Autodesk Inventor part; units mm, degrees
(part 6 of 6)
  arc A568 (-14.0614, 14.9173) -> (-13.8819, 14.463) centre (-6.919, 17.4773) ccw projected
  arc A569 (-13.7681, 15.1885) -> (-14.0614, 14.9173) centre (0, 0) ccw projected
  arc A570 (-13.3293, 14.9739) -> (-13.7681, 15.1885) centre (-16.8806, 8.2689) ccw projected
  arc A571 (-12.9866, 14.7786) -> (-13.3293, 14.9739) centre (-16.3285, 9.3114) ccw projected
  arc A572 (-12.7266, 14.609) -> (-12.9866, 14.7786) centre (-15.7361, 10.2805) ccw projected
  arc A573 (-12.4383, 14.8553) -> (-12.7266, 14.609) centre (0, 0) ccw projected
  arc A574 (-12.5651, 15.1386) -> (-12.4383, 14.8553) centre (-7.6922, 17.1506) ccw projected
  arc A575 (-12.7043, 15.5076) -> (-12.5651, 15.1386) centre (-6.6424, 17.5841) ccw projected
  arc A576 (-12.8477, 15.9746) -> (-12.7043, 15.5076) centre (-5.5264, 17.9663) ccw projected
  arc A577 (-12.534, 16.2219) -> (-12.8477, 15.9746) centre (0, 0) ccw projected
  arc A578 (-12.1134, 15.9735) -> (-12.534, 16.2219) centre (-16.1798, 9.5679) ccw projected
  arc A579 (-11.7871, 15.752) -> (-12.1134, 15.9735) centre (-15.5476, 10.5638) ccw projected
  arc A580 (-11.5412, 15.5625) -> (-11.7871, 15.752) centre (-14.881, 11.4834) ccw projected
  arc A581 (-11.2344, 15.7854) -> (-11.5412, 15.5625) centre (0, 0) ccw projected
  arc A582 (-11.3386, 16.0778) -> (-11.2344, 15.7854) centre (-6.3229, 17.7012) ccw projected
  arc A583 (-11.4485, 16.4566) -> (-11.3386, 16.0778) centre (-5.2423, 18.051) ccw projected
  arc A584 (-11.5547, 16.9334) -> (-11.4485, 16.4566) centre (-4.0998, 18.3445) ccw projected
  arc A585 (-11.2226, 17.1553) -> (-11.5547, 16.9334) centre (0, 0) ccw projected
  arc A586 (-10.8227, 16.8747) -> (-11.2226, 17.1553) centre (-15.3792, 10.8078) ccw projected
  arc A587 (-10.5148, 16.6282) -> (-10.8227, 16.8747) centre (-14.6708, 11.7511) ccw projected
  arc A588 (-10.2846, 16.42) -> (-10.5148, 16.6282) centre (-13.9341, 12.6156) ccw projected
  arc A589 (-9.9612, 16.6182) -> (-10.2846, 16.42) centre (0, 0) ccw projected
  arc A590 (-10.0422, 16.9178) -> (-9.9612, 16.6182) centre (-4.9146, 18.1428) ccw projected
  arc A591 (-10.122, 17.3041) -> (-10.0422, 16.9178) centre (-3.8099, 18.4067) ccw projected
  arc A592 (-10.1905, 17.7877) -> (-10.122, 17.3041) centre (-2.6478, 18.6096) ccw projected
  arc A593 (-9.842, 17.9829) -> (-10.1905, 17.7877) centre (0, 0) ccw projected
  arc A594 (-9.4654, 17.6718) -> (-9.842, 17.9829) centre (-14.4838, 11.9812) ccw projected
  arc A595 (-9.1778, 17.4019) -> (-9.4654, 17.6718) centre (-13.7036, 12.8659) ccw projected
  arc A596 (-8.9646, 17.1763) -> (-9.1778, 17.4019) centre (-12.9014, 13.6699) ccw projected
  arc A597 (-8.6267, 17.3485) -> (-8.9646, 17.1763) centre (0, 0) ccw projected
  arc A598 (-8.6839, 17.6536) -> (-8.6267, 17.3485) centre (-3.476, 18.4724) ccw projected
  arc A599 (-8.7331, 18.0449) -> (-8.6839, 17.6536) centre (-2.3539, 18.6488) ccw projected
  arc A600 (-8.7635, 18.5324) -> (-8.7331, 18.0449) centre (-1.1796, 18.76) ccw projected
  arc A601 (-8.4007, 18.6997) -> (-8.7635, 18.5324) centre (0, 0) ccw projected
  arc A602 (-8.0497, 18.36) -> (-8.4007, 18.6997) centre (-13.4991, 13.0806) ccw projected
  arc A603 (-7.7842, 18.0684) -> (-8.0497, 18.36) centre (-12.6519, 13.9014) ccw projected
  arc A604 (-7.5893, 17.8267) -> (-7.7842, 18.0684) centre (-11.7891, 14.64) ccw projected
  arc A605 (-7.2389, 17.9719) -> (-7.5893, 17.8267) centre (0, 0) ccw projected
  arc A606 (-7.272, 18.2805) -> (-7.2389, 17.9719) centre (-2.0159, 18.6882) ccw projected
  arc A607 (-7.2904, 18.6745) -> (-7.272, 18.2805) centre (-0.8835, 18.776) ccw projected
  arc A608 (-7.2825, 19.1629) -> (-7.2904, 18.6745) centre (0.2959, 18.7947) ccw projected
  arc A609 (-6.9077, 19.3011) -> (-7.2825, 19.1629) centre (0, 0) ccw projected
  arc A610 (-6.5844, 18.9349) -> (-6.9077, 19.3011) centre (-12.4312, 14.0994) ccw projected
  arc A611 (-6.3425, 18.6234) -> (-6.5844, 18.9349) centre (-11.5222, 14.8512) ccw projected
  arc A612 (-6.1673, 18.3672) -> (-6.3425, 18.6234) centre (-10.6041, 15.5199) ccw projected
  arc A613 (-5.8066, 18.4844) -> (-6.1673, 18.3672) centre (0, 0) ccw projected
  arc A614 (-5.8154, 18.7947) -> (-5.8066, 18.4844) centre (-0.5434, 18.7888) ccw projected
  arc A615 (-5.8028, 19.1889) -> (-5.8154, 18.7947) centre (0.5924, 18.7875) ccw projected
  arc A616 (-5.7565, 19.6752) -> (-5.8028, 19.1889) centre (1.7696, 18.7136) ccw projected
  arc A617 (-5.372, 19.7836) -> (-5.7565, 19.6752) centre (0, 0) ccw projected
  arc A618 (-5.0785, 19.3932) -> (-5.372, 19.7836) centre (-11.2867, 15.0313) ccw projected
  arc A619 (-4.8618, 19.0636) -> (-5.0785, 19.3932) centre (-10.3215, 15.7095) ccw projected
  arc A620 (-4.7072, 18.7945) -> (-4.8618, 19.0636) centre (-9.3537, 16.304) ccw projected
  arc A621 (-4.3384, 18.883) -> (-4.7072, 18.7945) centre (0, 0) ccw projected
  arc A622 (-4.3228, 19.193) -> (-4.3384, 18.883) centre (0.9324, 18.7735) ccw projected
  arc A623 (-4.2793, 19.585) -> (-4.3228, 19.193) centre (2.0646, 18.6831) ccw projected
  arc A624 (-4.1951, 20.0662) -> (-4.2793, 19.585) centre (3.2324, 18.517) ccw projected
  arc A625 (-3.8033, 20.1441) -> (-4.1951, 20.0662) centre (0, 0) ccw projected
  arc A626 (-3.5413, 19.7318) -> (-3.8033, 20.1441) centre (-10.0726, 15.8705) ccw projected
  arc A627 (-3.3511, 19.3863) -> (-3.5413, 19.7318) centre (-9.0571, 16.4708) ccw projected
  arc A628 (-3.2181, 19.1059) -> (-3.3511, 19.3863) centre (-8.0457, 16.9876) ccw projected
  arc A629 (-2.8435, 19.1652) -> (-3.2181, 19.1059) centre (0, 0) ccw projected
  arc A630 (-2.8036, 19.473) -> (-2.8435, 19.1652) centre (2.4025, 18.6425) ccw projected
  arc A631 (-2.7295, 19.8604) -> (-2.8036, 19.473) centre (3.5241, 18.4635) ccw projected
  arc A632 (-2.6078, 20.3335) -> (-2.7295, 19.8604) centre (4.6753, 18.2064) ccw projected
  arc A633 (-2.2111, 20.3804) -> (-2.6078, 20.3335) centre (0, 0) ccw projected
  arc A634 (-1.9822, 19.9489) -> (-2.2111, 20.3804) centre (-8.7963, 16.6119) ccw projected
  arc A635 (-1.8197, 19.5895) -> (-1.9822, 19.9489) centre (-7.7369, 17.1307) ccw projected
  arc A636 (-1.7091, 19.2995) -> (-1.8197, 19.5895) centre (-6.6881, 17.5665) ccw projected
  arc A637 (-1.331, 19.3292) -> (-1.7091, 19.2995) centre (0, 0) ccw projected
  arc A638 (-1.2671, 19.633) -> (-1.331, 19.3292) centre (3.8577, 18.3965) ccw projected
  arc A639 (-1.1629, 20.0133) -> (-1.2671, 19.633) centre (4.9618, 18.1301) ccw projected
  arc A640 (-1.0044, 20.4754) -> (-1.1629, 20.0133) centre (6.0894, 17.7834) ccw projected
  arc A641 (-0.6052, 20.4911) -> (-1.0044, 20.4754) centre (0, 0) ccw projected
  arc A642 (-0.4109, 20.0429) -> (-0.6052, 20.4911) centre (-7.4658, 17.2508) ccw projected
  circle A643 centre (0, 0) radius 18.25 projected
  line L0 (-18.25, 0) -> (18.25, 0) construction
  arc A644 (-18.25, 2.5) -> (-18.25, -2.5) centre (-18.25, 0) ccw
  arc A645 (18.25, -2.5) -> (18.25, 2.5) centre (18.25, 0) ccw
  line L1 (0, 18.25) -> (0, -18.25) construction
  arc A646 (2.5, 18.25) -> (-2.5, 18.25) centre (0, 18.25) ccw
  arc A647 (-2.5, -18.25) -> (2.5, -18.25) centre (0, -18.25) ccw
  line L2 (-18.25, -2.5) -> (-18.078, -2.5)
  arc A648 (-14.7902, -2.5) -> (-2.5, -14.7902) centre (0, 0) ccw
  line L3 (-2.5, -18.078) -> (-2.5, -18.25)
  line L4 (2.5, -18.25) -> (2.5, -18.078)
  arc A649 (2.5, -14.7902) -> (14.7902, -2.5) centre (0, 0) ccw
  line L5 (18.078, -2.5) -> (18.25, -2.5)
  line L6 (18.25, 2.5) -> (18.078, 2.5)
  arc A650 (14.7902, 2.5) -> (2.5, 14.7902) centre (0, 0) ccw
  arc A651 (-2.5, 14.7902) -> (-14.7902, 2.5) centre (0, 0) ccw
  line L7 (2.5, 18.078) -> (2.5, 18.25)
  line L8 (-2.5, 18.25) -> (-2.5, 18.078)
  line L9 (-18.078, 2.5) -> (-18.25, 2.5)
  line L10 (-14.7902, -2.5) -> (-5.4544, -2.5)
  line L11 (-2.5, -5.4544) -> (-2.5, -14.7902)
  line L12 (2.5, -14.7902) -> (2.5, -5.4544)
  line L13 (-2.5, -2.5) -> (2.5, -2.5)
  line L14 (5.4544, -2.5) -> (14.7902, -2.5)
  line L15 (14.7902, 2.5) -> (5.4544, 2.5)
  line L16 (2.5, -2.5) -> (2.5, 2.5)
  line L17 (2.5, 5.4544) -> (2.5, 14.7902)
  line L18 (-2.5, 14.7902) -> (-2.5, 5.4544)
  line L19 (-2.5, 2.5) -> (-2.5, -2.5)
  line L20 (2.5, 2.5) -> (-2.5, 2.5)
  line L21 (-5.4544, 2.5) -> (-14.7902, 2.5)
  point P0 (148.5, -105)
  dimension "d20" = 5
  dimension "d21" = 5
  constraints: 50 parallel, 48 end point, 40 tangent, 20 point on circle, 8 centre point, 4 midpoint, 1 coincident, 1 horizontal, 1 vertical, 22 other
  measures "d20" diameter of A645
  measures "d21" diameter of A647
extrude "押し出し5" cut sketch "スケッチ5" against normal blind 10 contours A0 L17 A650 L15 | L14 A649 L12 A0 | A0 L21 A651 L18 | L11 A648 L10 A0
fillet "フィレット2" radius 1 8 edges at (163.2902, 102.5, 1.5) (163.2902, 107.5, 1.5) (151, 119.7902, 1.5) (146, 119.7902, 1.5) (146, 90.2098, 1.5) (151, 90.2098, 1.5) (133.7098, 102.5, 1.5) (133.7098, 107.5, 1.5)
fillet "フィレット3" radius 5 8 edges at (153.9544, 102.5, 1.5) (153.9544, 107.5, 1.5) (151, 99.5456, 1.5) (146, 99.5456, 1.5) (143.0456, 102.5, 1.5) (143.0456, 107.5, 1.5) (146, 110.4544, 1.5) (151, 110.4544, 1.5)
sketch "スケッチ6" plane through (0, 0, -5) normal (0, 0, -1) x (-1, 0, 0)
  circle A0 centre (-148.5, 105) radius 2 projected
  arc A1 (-149.1615, 109.6213) -> (-149.1982, 109.7586) centre (-149.7545, 109.5365) ccw projected
  arc A2 (-149.1982, 109.7586) -> (-149.402, 110.1264) centre (-150.7515, 109.1382) ccw projected
  arc A3 (-149.402, 110.1264) -> (-150.0725, 110.7903) centre (-151.8157, 108.3591) ccw projected
  arc A4 (-150.0725, 110.7903) -> (-150.6312, 110.6087) centre (-148.5, 105) ccw projected
  arc A5 (-150.6312, 110.6087) -> (-150.7841, 109.6791) centre (-147.7926, 109.6645) ccw projected
  arc A6 (-150.7841, 109.6791) -> (-150.7328, 109.2599) centre (-149.1115, 109.671) ccw projected
  arc A7 (-150.7328, 109.2599) -> (-150.6818, 109.1272) centre (-150.1522, 109.4071) ccw projected
  line L0 (-150.6818, 109.1272) -> (-150.4726, 108.7315) projected
  arc A8 (-150.6306, 108.0863) -> (-150.4726, 108.7315) centre (-150.9147, 108.4978) ccw projected
  arc A9 (-150.6306, 108.0863) -> (-150.7779, 107.9793) centre (-148.5, 105) ccw projected
  arc A10 (-151.4403, 108.0283) -> (-150.7779, 107.9793) centre (-151.0815, 108.3766) ccw projected
  line L1 (-151.4403, 108.0283) -> (-151.7519, 108.3493) projected
  arc A11 (-151.7519, 108.3493) -> (-151.8623, 108.4388) centre (-152.1817, 107.9321) ccw projected
  arc A12 (-151.8623, 108.4388) -> (-152.2451, 108.6171) centre (-152.7543, 107.0239) ccw projected
  arc A13 (-152.2451, 108.6171) -> (-153.1765, 108.759) centre (-153.1557, 105.7676) ccw projected
  arc A14 (-153.1765, 108.759) -> (-153.5209, 108.2848) centre (-148.5, 105) ccw projected
  arc A15 (-153.5209, 108.2848) -> (-153.0982, 107.4429) centre (-150.6695, 109.1895) ccw projected
  arc A16 (-153.0982, 107.4429) -> (-152.8103, 107.1339) centre (-151.7402, 108.4195) ccw projected
  arc A17 (-152.8103, 107.1339) -> (-152.691, 107.0565) centre (-152.4271, 107.5943) ccw projected
  line L2 (-152.691, 107.0565) -> (-152.2892, 106.8594) projected
  arc A18 (-152.0378, 106.2446) -> (-152.2892, 106.8594) centre (-152.5095, 106.4105) ccw projected
  arc A19 (-152.0378, 106.2446) -> (-152.094, 106.0715) centre (-148.5, 105) ccw projected
  arc A20 (-152.6588, 105.7217) -> (-152.094, 106.0715) centre (-152.5732, 106.2143) ccw projected
  line L3 (-152.6588, 105.7217) -> (-153.0995, 105.7982) projected
  arc A21 (-153.0995, 105.7982) -> (-153.2414, 105.8058) centre (-153.202, 105.2081) ccw projected
  arc A22 (-153.2414, 105.8058) -> (-153.656, 105.725) centre (-153.1314, 104.1367) ccw projected
  arc A23 (-153.656, 105.725) -> (-154.4929, 105.2923) centre (-152.7177, 102.8844) ccw projected
  arc A24 (-154.4929, 105.2923) -> (-154.4928, 104.7063) centre (-148.5, 105) ccw projected
  arc A25 (-154.4928, 104.7063) -> (-153.6559, 104.2736) centre (-152.7177, 107.1142) ccw projected
  arc A26 (-153.6559, 104.2736) -> (-153.2414, 104.1928) centre (-153.1313, 105.8619) ccw projected
  arc A27 (-153.2414, 104.1928) -> (-153.0993, 104.2004) centre (-153.2019, 104.7905) ccw projected
  line L4 (-153.0993, 104.2004) -> (-152.6585, 104.277) projected
  arc A28 (-152.0937, 103.9274) -> (-152.6585, 104.277) centre (-152.5728, 103.7844) ccw projected
  arc A29 (-152.0937, 103.9274) -> (-152.0374, 103.7543) centre (-148.5, 105) ccw projected
  arc A30 (-152.2887, 103.1394) -> (-152.0374, 103.7543) centre (-152.509, 103.5882) ccw projected
  line L5 (-152.2887, 103.1394) -> (-152.6903, 102.9423) projected
  arc A31 (-152.6903, 102.9423) -> (-152.8095, 102.8649) centre (-152.4263, 102.4046) ccw projected
  arc A32 (-152.8095, 102.8649) -> (-153.0974, 102.5559) centre (-151.7394, 101.5794) ccw projected
  arc A33 (-153.0974, 102.5559) -> (-153.5202, 101.714) centre (-150.6687, 100.8093) ccw projected
  arc A34 (-153.5202, 101.714) -> (-153.1756, 101.2399) centre (-148.5, 105) ccw projected
  arc A35 (-153.1756, 101.2399) -> (-152.2442, 101.3818) centre (-153.1548, 104.2313) ccw projected
  arc A36 (-152.2442, 101.3818) -> (-151.8614, 101.5601) centre (-152.7534, 102.9751) ccw projected
  arc A37 (-151.8614, 101.5601) -> (-151.7509, 101.6497) centre (-152.1808, 102.0668) ccw projected
  line L6 (-151.7509, 101.6497) -> (-151.4393, 101.9708) projected
  arc A38 (-150.7769, 102.0199) -> (-151.4393, 101.9708) centre (-151.0805, 101.6226) ccw projected
  arc A39 (-150.7769, 102.0199) -> (-150.6296, 101.913) centre (-148.5, 105) ccw projected
  arc A40 (-150.4715, 101.2678) -> (-150.6296, 101.913) centre (-150.9136, 101.5014) ccw projected
  line L7 (-150.4715, 101.2678) -> (-150.6805, 100.8723) projected
  arc A41 (-150.6805, 100.8723) -> (-150.7315, 100.7396) centre (-150.1509, 100.5924) ccw projected
  arc A42 (-150.7315, 100.7396) -> (-150.7828, 100.3204) centre (-149.1102, 100.3285) ccw projected
  arc A43 (-150.7828, 100.3204) -> (-150.6299, 99.3908) centre (-147.7913, 100.335) ccw projected
  arc A44 (-150.6299, 99.3908) -> (-150.0725, 99.2097) centre (-148.5, 105) ccw projected
  arc A45 (-150.0725, 99.2097) -> (-149.4024, 99.872) centre (-151.814, 101.6421) ccw projected
  arc A46 (-149.4024, 99.872) -> (-149.1975, 100.2413) centre (-150.7508, 100.8617) ccw projected
  arc A47 (-149.1975, 100.2413) -> (-149.1608, 100.3787) centre (-149.7538, 100.4635) ccw projected
  line L8 (-149.1608, 100.3787) -> (-149.0974, 100.8217) projected
  arc A48 (-148.5904, 101.2507) -> (-149.0974, 100.8217) centre (-148.6025, 100.7509) ccw projected
  arc A49 (-148.5904, 101.2507) -> (-148.409, 101.2508) centre (-148.5, 105) ccw projected
  arc A50 (-147.9019, 100.8217) -> (-148.409, 101.2508) centre (-148.3969, 100.7509) ccw projected
  line L9 (-147.9019, 100.8217) -> (-147.8385, 100.3788) projected
  arc A51 (-147.8385, 100.3788) -> (-147.8018, 100.2415) centre (-147.2456, 100.4636) ccw projected
  arc A52 (-147.8018, 100.2415) -> (-147.5969, 99.8722) centre (-146.2485, 100.8619) ccw projected
  arc A53 (-147.5969, 99.8722) -> (-146.9268, 99.2099) centre (-145.1853, 101.6423) ccw projected
  arc A54 (-146.9268, 99.2099) -> (-146.3695, 99.391) centre (-148.5, 105) ccw projected
  arc A55 (-146.3695, 99.391) -> (-146.2166, 100.3207) centre (-149.2081, 100.3352) ccw projected
  arc A56 (-146.2166, 100.3207) -> (-146.2679, 100.7399) centre (-147.8892, 100.3288) ccw projected
  arc A57 (-146.2679, 100.7399) -> (-146.3189, 100.8726) centre (-146.8485, 100.5927) ccw projected
  line L10 (-146.3189, 100.8726) -> (-146.528, 101.2681) projected
  arc A58 (-146.3699, 101.9133) -> (-146.528, 101.2681) centre (-146.0859, 101.5018) ccw projected
  arc A59 (-146.3699, 101.9133) -> (-146.2231, 102.0199) centre (-148.5, 105) ccw projected
  arc A60 (-145.5608, 101.9708) -> (-146.2231, 102.0199) centre (-145.9196, 101.6226) ccw projected
  line L11 (-145.5608, 101.9708) -> (-145.249, 101.6496) projected
  arc A61 (-145.249, 101.6496) -> (-145.1386, 101.5601) centre (-144.8192, 102.0668) ccw projected
  arc A62 (-145.1386, 101.5601) -> (-144.7558, 101.3818) centre (-144.2466, 102.9751) ccw projected
  arc A63 (-144.7558, 101.3818) -> (-143.8244, 101.2399) centre (-143.8452, 104.2313) ccw projected
  arc A64 (-143.8244, 101.2399) -> (-143.4791, 101.7152) centre (-148.5, 105) ccw projected
  arc A65 (-143.4791, 101.7152) -> (-143.9018, 102.5571) centre (-146.3305, 100.8105) ccw projected
  arc A66 (-143.9018, 102.5571) -> (-144.1897, 102.8661) centre (-145.2598, 101.5805) ccw projected
  arc A67 (-144.1897, 102.8661) -> (-144.309, 102.9435) centre (-144.5729, 102.4057) ccw projected
  line L12 (-144.309, 102.9435) -> (-144.7108, 103.1406) projected
  arc A68 (-144.9622, 103.7554) -> (-144.7108, 103.1406) centre (-144.4905, 103.5895) ccw projected
  arc A69 (-144.9622, 103.7554) -> (-144.9063, 103.9274) centre (-148.5, 105) ccw projected
  arc A70 (-144.3416, 104.277) -> (-144.9063, 103.9274) centre (-144.4272, 103.7844) ccw projected
  line L13 (-144.3416, 104.277) -> (-143.9006, 104.2004) projected
  arc A71 (-143.9006, 104.2004) -> (-143.7586, 104.1928) centre (-143.7981, 104.7905) ccw projected
  arc A72 (-143.7586, 104.1928) -> (-143.3441, 104.2736) centre (-143.8687, 105.8619) ccw projected
  arc A73 (-143.3441, 104.2736) -> (-142.5072, 104.7063) centre (-144.2823, 107.1142) ccw projected
  arc A74 (-142.5072, 104.7063) -> (-142.5072, 105.2937) centre (-148.5, 105) ccw projected
  arc A75 (-142.5072, 105.2937) -> (-143.3441, 105.7264) centre (-144.2823, 102.8858) ccw projected
  arc A76 (-143.3441, 105.7264) -> (-143.7586, 105.8072) centre (-143.8687, 104.1381) ccw projected
  arc A77 (-143.7586, 105.8072) -> (-143.9007, 105.7996) centre (-143.7981, 105.2095) ccw projected
  line L14 (-143.9007, 105.7996) -> (-144.3415, 105.723) projected
  arc A78 (-144.9063, 106.0726) -> (-144.3415, 105.723) centre (-144.4272, 106.2156) ccw projected
  arc A79 (-144.9063, 106.0726) -> (-144.9622, 106.2445) centre (-148.5, 105) ccw projected
  arc A80 (-144.7108, 106.8593) -> (-144.9622, 106.2445) centre (-144.4905, 106.4104) ccw projected
  line L15 (-144.7108, 106.8593) -> (-144.309, 107.0566) projected
  arc A81 (-144.309, 107.0566) -> (-144.1897, 107.1339) centre (-144.5729, 107.5943) ccw projected
  arc A82 (-144.1897, 107.1339) -> (-143.9018, 107.4429) centre (-145.2598, 108.4195) ccw projected
  arc A83 (-143.9018, 107.4429) -> (-143.4791, 108.2848) centre (-146.3305, 109.1895) ccw projected
  arc A84 (-143.4791, 108.2848) -> (-143.8244, 108.7601) centre (-148.5, 105) ccw projected
  arc A85 (-143.8244, 108.7601) -> (-144.7558, 108.6182) centre (-143.8452, 105.7687) ccw projected
  arc A86 (-144.7558, 108.6182) -> (-145.1386, 108.4399) centre (-144.2466, 107.0249) ccw projected
  arc A87 (-145.1386, 108.4399) -> (-145.2491, 108.3503) centre (-144.8192, 107.9332) ccw projected
  line L16 (-145.2491, 108.3503) -> (-145.5607, 108.0292) projected
  arc A88 (-146.2231, 107.9801) -> (-145.5607, 108.0292) centre (-145.9195, 108.3774) ccw projected
  arc A89 (-146.2231, 107.9801) -> (-146.3693, 108.0863) centre (-148.5, 105) ccw projected
  arc A90 (-146.5274, 108.7314) -> (-146.3693, 108.0863) centre (-146.0853, 108.4978) ccw projected
  line L17 (-146.5274, 108.7314) -> (-146.3182, 109.1272) projected
  arc A91 (-146.3182, 109.1272) -> (-146.2672, 109.2599) centre (-146.8478, 109.4071) ccw projected
  arc A92 (-146.2672, 109.2599) -> (-146.2159, 109.6791) centre (-147.8885, 109.671) ccw projected
  arc A93 (-146.2159, 109.6791) -> (-146.3688, 110.6087) centre (-149.2074, 109.6645) ccw projected
  arc A94 (-146.3688, 110.6087) -> (-146.9275, 110.7903) centre (-148.5, 105) ccw projected
  arc A95 (-146.9275, 110.7903) -> (-147.5976, 110.128) centre (-145.186, 108.3579) ccw projected
  arc A96 (-147.5976, 110.128) -> (-147.8025, 109.7587) centre (-146.2492, 109.1383) ccw projected
  arc A97 (-147.8025, 109.7587) -> (-147.8392, 109.6213) centre (-147.2462, 109.5365) ccw projected
  line L18 (-147.8392, 109.6213) -> (-147.9026, 109.1783) projected
  arc A98 (-148.4096, 108.7493) -> (-147.9026, 109.1783) centre (-148.3975, 109.2491) ccw projected
  arc A99 (-148.4096, 108.7493) -> (-148.591, 108.7492) centre (-148.5, 105) ccw projected
  arc A100 (-149.0981, 109.1783) -> (-148.591, 108.7492) centre (-148.6031, 109.2491) ccw projected
  line L19 (-149.0981, 109.1783) -> (-149.1615, 109.6213) projected
  line L20 (-146, 91.4446) -> (-146, 96.9533) projected
  arc A101 (-144.4091, 100.6109) -> (-146, 96.9533) centre (-141, 96.9533) ccw projected
  arc A102 (-152.5909, 100.6109) -> (-144.4091, 100.6109) centre (-148.5, 105) ccw projected
  arc A103 (-151, 96.9533) -> (-152.5909, 100.6109) centre (-156, 96.9533) ccw projected
  line L21 (-151, 96.9533) -> (-151, 91.4446) projected
  arc A104 (-152.25, 90.4763) -> (-151, 91.4446) centre (-152, 91.4446) ccw projected
  arc A105 (-163.0237, 101.25) -> (-152.25, 90.4763) centre (-148.5, 105) ccw projected
  arc A106 (-162.0554, 102.5) -> (-163.0237, 101.25) centre (-162.0554, 101.5) ccw projected
  line L22 (-162.0554, 102.5) -> (-156.5467, 102.5) projected
  arc A107 (-152.8891, 100.9091) -> (-156.5467, 102.5) centre (-156.5467, 97.5) ccw projected
  arc A108 (-152.8891, 109.0909) -> (-152.8891, 100.9091) centre (-148.5, 105) ccw projected
  arc A109 (-156.5467, 107.5) -> (-152.8891, 109.0909) centre (-156.5467, 112.5) ccw projected
  line L23 (-156.5467, 107.5) -> (-162.0554, 107.5) projected
  arc A110 (-163.0237, 108.75) -> (-162.0554, 107.5) centre (-162.0554, 108.5) ccw projected
  arc A111 (-152.25, 119.5237) -> (-163.0237, 108.75) centre (-148.5, 105) ccw projected
  arc A112 (-151, 118.5554) -> (-152.25, 119.5237) centre (-152, 118.5554) ccw projected
  line L24 (-151, 118.5554) -> (-151, 113.0467) projected
  arc A113 (-152.5909, 109.3891) -> (-151, 113.0467) centre (-156, 113.0467) ccw projected
  arc A114 (-144.4091, 109.3891) -> (-152.5909, 109.3891) centre (-148.5, 105) ccw projected
  arc A115 (-146, 113.0467) -> (-144.4091, 109.3891) centre (-141, 113.0467) ccw projected
  line L25 (-146, 113.0467) -> (-146, 118.5554) projected
  arc A116 (-144.75, 119.5237) -> (-146, 118.5554) centre (-145, 118.5554) ccw projected
  arc A117 (-133.9763, 108.75) -> (-144.75, 119.5237) centre (-148.5, 105) ccw projected
  arc A118 (-134.9446, 107.5) -> (-133.9763, 108.75) centre (-134.9446, 108.5) ccw projected
  line L26 (-134.9446, 107.5) -> (-140.4533, 107.5) projected
  arc A119 (-144.1109, 109.0909) -> (-140.4533, 107.5) centre (-140.4533, 112.5) ccw projected
  arc A120 (-144.1109, 100.9091) -> (-144.1109, 109.0909) centre (-148.5, 105) ccw projected
  arc A121 (-140.4533, 102.5) -> (-144.1109, 100.9091) centre (-140.4533, 97.5) ccw projected
  line L27 (-140.4533, 102.5) -> (-134.9446, 102.5) projected
  arc A122 (-133.9763, 101.25) -> (-134.9446, 102.5) centre (-134.9446, 101.5) ccw projected
  arc A123 (-144.75, 90.4763) -> (-133.9763, 101.25) centre (-148.5, 105) ccw projected
  arc A124 (-146, 91.4446) -> (-144.75, 90.4763) centre (-145, 91.4446) ccw projected
  circle A125 centre (-148.5, 105) radius 18.25 projected
  circle A126 centre (-148.5, 105) radius 6
  point P0 (0, 0)
  constraints: 1 coincident, 3 other
